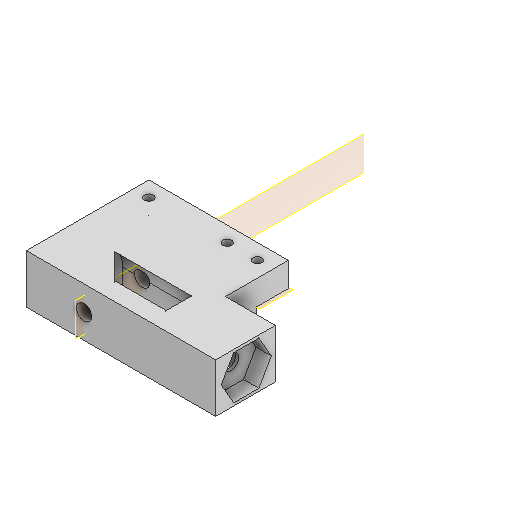
# Autodesk Inventor part: 30_Lightsheet_generator_passive_lid_v0
Saved by Autodesk Inventor 2022 (Build 260153000, 153)
## iProperties
Created: 2022-12-16
Part Number: 30_Lightsheet_generator_passive_lid_v0
Material: Generisch
Document SubType Name: Modeling
Designer: UC2
Density: 1 g/cm^3
Appearance: Vorgabe
Author: UC2
Autodesk Inventor part; units mm, degrees
ref_plane "Arbeitsebene6" through (18.9, 3.95, -31.1) normal (0, 1, 0) x (-1, 0, 0)
sketch "Skizze13" plane through (18.9, 3.95, -31.1) normal (0, 1, 0) x (-1, 0, 0)
  circle A0 centre (40.5, 5) radius 1.45 projected
  line L0 (29.1796, 0.9) -> (29.1796, 0) projected
  line L1 (45.5, 0) -> (29.1796, 0) projected
  line L2 (45.5, 0) -> (45.5, 10) projected
  line L3 (45.5, 10) -> (29.1796, 10) projected
  line L4 (29.1796, 10) -> (29.1796, 6.8717) projected
  line L5 (29.1796, 6.8717) -> (32.9296, 6.8717) projected
  line L6 (32.9296, 6.8717) -> (32.9296, 0.9) projected
  line L7 (32.9296, 0.9) -> (29.1796, 0.9) projected
  line L8 (24.1796, 0) -> (24.1796, 0.9) projected
  line L9 (24.1796, 0.9) -> (20.4296, 0.9) projected
  line L10 (20.4296, 0.9) -> (20.4296, 6.8717) projected
  line L11 (20.4296, 6.8717) -> (24.1796, 6.8717) projected
  line L12 (24.1796, 6.8717) -> (24.1796, 10) projected
  line L13 (24.1796, 10) -> (0, 10) projected
  line L14 (0, 0) -> (0, 10) projected
  line L15 (24.1796, 0) -> (0, 0) projected
  circle A1 centre (14.9199, 5) radius 1.45 projected
  circle A2 centre (5.0801, 5) radius 1.45 projected
  line L16 (29.1796, 10) -> (24.1796, 10)
  line L17 (29.1796, 0) -> (24.1796, 0)
  line L18 (55.5, 0) -> (55.5, 10) projected
  line L19 (55.5, 10) -> (55.473, 10) projected
  line L20 (55.473, 10) -> (55.473, 40) projected
  line L21 (55.473, 40) -> (45.5, 40) projected
  line L22 (45.5, 40) -> (45.5, 20) projected
  line L23 (45.5, 20) -> (35.5, 20) projected
  line L24 (35.5, 20) -> (35.5, 10.0274) projected
  arc A3 (35.5, 10.0274) -> (35.527, 10) centre (40.5, 14.9264) ccw projected
  line L25 (45.5, 10) -> (35.527, 10) projected
  line L26 (45.5, 0) -> (45.5, 10) projected
  line L27 (45.5, 0) -> (55.5, 0) projected
  line L28 (52.073, 16.5) -> (52.073, 3.5) projected
  arc A4 (48.873, 3.5) -> (52.073, 3.5) centre (50.473, 3.5) ccw projected
  line L29 (48.873, 3.5) -> (48.873, 16.5) projected
  arc A5 (52.073, 16.5) -> (48.873, 16.5) centre (50.473, 16.5) ccw projected
  line L30 (48.8865, 23.1111) -> (48.8865, 36.1111) projected
  arc A6 (52.0865, 36.1111) -> (48.8865, 36.1111) centre (50.4865, 36.1111) ccw projected
  line L31 (52.0865, 36.1111) -> (52.0865, 23.1111) projected
  arc A7 (48.8865, 23.1111) -> (52.0865, 23.1111) centre (50.4865, 23.1111) ccw projected
  line L32 (-10, 0) -> (0, 0) projected
  line L33 (0, 10) -> (0, 0) projected
  line L34 (16, 10) -> (0, 10) projected
  line L35 (16, 10) -> (16, 20) projected
  line L36 (16, 20) -> (-10, 20) projected
  line L37 (-10, 20) -> (-10, 0) projected
  line L38 (-3.4, 16.5) -> (-3.4, 3.5) projected
  arc A8 (-6.6, 3.5) -> (-3.4, 3.5) centre (-5, 3.5) ccw projected
  line L39 (-6.6, 3.5) -> (-6.6, 16.5) projected
  arc A9 (-3.4, 16.5) -> (-6.6, 16.5) centre (-5, 16.5) ccw projected
  line L40 (-16.2879, 40) -> (45.5, 40)
  line L41 (45.5, 40) -> (45.5, 20.5)
  line L42 (45.5, 20.5) -> (-16.2879, 20.5)
  line L43 (-16.2879, 20.5) -> (-16.2879, 40)
  line L44 (45.5, 20.5) -> (35.5, 20.5)
  line L45 (35.5, 20.5) -> (35.5, 20)
  line L46 (35.5, 20) -> (45.5, 20)
  line L47 (45.5, 20) -> (45.5, 20.5)
  line L48 (16, 20) -> (0, 20)
  line L49 (0, 20) -> (0, 20.5)
  line L50 (0, 20.5) -> (16, 20.5)
  line L51 (16, 20.5) -> (16, 20)
  line L52 (0, 20) -> (0, 10)
  line L53 (35.5, 10) -> (45.5, 10)
  line L54 (45.5, 10) -> (45.5, 20.5)
  line L55 (45.5, 20.5) -> (35.5, 20.5)
  line L56 (35.5, 20.5) -> (35.5, 10)
  point P0 (0, 20)
  point P1 (0.5252, 10)
  point P2 (35.527, 10)
  point P3 (0, 20)
  point P4 (35.5, 10.0274)
  dimension "d60" = 0.5
  constraints: 38 end point, 9 parallel, 5 horizontal, 5 perpendicular, 3 point on line
  measures "d60" distance between parallel lines of L23 L42
extrude "Extrusion12" add sketch "Skizze13" along normal blind 8 contours L7 L6 L5 L4 L3 L2 L1 L0 | L0 L17 L8 L9 L10 L11 L12 L16 L4 L5 L6 L7 | L15 L14 L13 L12 L11 L10 L9 L8 | L3 A3 L24 L23 L54 | L23 L45 L42 L22 | L52 L36 L35 L13 | L16 L13 L35 L51 L42 L45 L24 L56 L3 | L42 L43 L40 L22 | L49 L42 L51 L36
sketch "Skizze16" plane through (18.9, 3.95, -31.1) normal (0, -1, 0) x (1, 0, 0)
  line L0 (16.2879, 20.5) -> (0, 20.5) projected
  line L1 (-45.5, 0) -> (-45.5, 40) projected
  circle A0 centre (-5.0801, 5) radius 1.45 projected
  circle A1 centre (-14.9199, 5) radius 1.45 projected
  line L2 (-16, 20) -> (10, 20) projected
  line L3 (-66.9798, -10.3003) -> (9.2505, 65.9301)
  line L4 (16.2879, 20.5) -> (0, 20.5) projected
  line L5 (16.2879, 20.5) -> (-45.5, 20.5)
  line L6 (-45.5, 20.5) -> (-45.5, 40)
  line L7 (-45.5, 40) -> (16.2879, 40)
  line L8 (16.2879, 40) -> (16.2879, 20.5)
  line L9 (0, 20.5) -> (0, 0) projected
  line L10 (16.2879, 40) -> (16.2879, 20.5) projected
  line L11 (-45.5, 40) -> (16.2879, 40) projected
  line L12 (0, 0) -> (-45.5, 0) projected
  point P0 (-18.9, 31.1)
  constraints: 10 end point, 2 parallel, 1 horizontal, 1 perpendicular, 3 other
extrude "Extrusion13" add sketch "Skizze16" along normal blind 8 contours L0 L5 L3 L7 L8 | L5 L1 L7 L3
ref_plane "Arbeitsebene7" through (-7.7796, -1.85, -37.9251) normal (1, 0, 0) x (0, -1, 0)
sketch "Skizze18" plane through (-7.7796, -1.85, -37.9251) normal (1, 0, 0) x (0, -1, 0)
  arc A0 (-5.8, -13.6968) -> (-0.7, -9.8391) centre (-5.8, -8.3968) ccw projected
  line L0 (-0.7, -9.8391) -> (-0.7, -7.7251) projected
  arc A1 (-10.8, -9.8251) -> (-0.8, -9.8251) centre (-5.8, -8.3968) ccw projected
  line L1 (-0.8, -7.8251) -> (-0.8, -9.8251) projected
  line L2 (-10.8, -7.8251) -> (-0.8, -7.8251) projected
  line L3 (-10.8, -9.8251) -> (-10.8, -7.8251) projected
  arc A2 (-10.9, -9.8391) -> (-0.7, -9.8391) centre (-5.8, -8.3968) ccw
  line L4 (-10.9, -9.8391) -> (-10.9, -7.7251)
  line L5 (-10.9, -7.7251) -> (-0.7, -7.7251)
  line L6 (-0.7, -7.7251) -> (-0.7, -9.8391)
  point P0 (-1.85, -37.9251)
  point P1 (-5.8, -13.6968)
  constraints: 6 end point, 2 point on circle, 1 centre point, 3 other
extrude "Extrusion15" cut sketch "Skizze18" along normal mid plane 12.5 contours A2 L4 L5 L0 A0 | L3 L2 L1 A1
sketch "Skizze19" plane through (35.1879, 11.95, 8.9) normal (1, 0, 0) x (0, 0, -1)
  circle A0 centre (10, -8) radius 7 projected
  circle A1 centre (10, -8) radius 7.1
  line L0 (14.0992, -15.1) -> (5.9008, -15.1)
  line L1 (5.9008, -15.1) -> (1.8016, -8)
  line L2 (1.8016, -8) -> (5.9008, -0.9)
  line L3 (5.9008, -0.9) -> (14.0992, -0.9)
  line L4 (14.0992, -0.9) -> (18.1984, -8)
  line L5 (18.1984, -8) -> (14.0992, -15.1)
  line L6 (19.5, -16) -> (0, -16) projected
  point P0 (8.9, -11.95)
  dimension "d68" = 0.1
  constraints: 12 end point, 1 centre point, 1 coincident, 1 parallel, 1 tangent, 13 other
  measures "d68" radial gap between concentric circles of A0 A1
ref_plane "Arbeitsebene8" through (22.1204, -2.15, -7.2) normal (1, 0, 0) x (0, 1, 0)
extrude "Extrusion16" cut sketch "Skizze19" against normal blind 5 contours A0 | A1 | A1 L4 L5 | A1 L3 L4 | L5 L0 A1 | A1 L2 L3 | L0 L1 A1 | A1 L1 L2
sketch "Skizze20" plane through (30.1879, 11.05, 2.9992) normal (1, 0, 0) x (0, 0, -1)
  arc A0 (6.1223, -12.104) -> (2.4773, -12.2481) centre (4.0992, -7.1) ccw projected
  circle A1 centre (4.0992, -7.1) radius 6.15
  line L0 (10.2492, -7.1) -> (-2.0508, -7.1)
  line L1 (-2.0508, -7.1) -> (-2.0508, -16.2052)
  line L2 (-2.0508, -16.2052) -> (10.2492, -16.2052)
  line L3 (10.2492, -16.2052) -> (10.2492, -7.1)
  point P0 (2.9992, -11.05)
  point P1 (-2.0508, -7.1)
  dimension "d71" = 12.3
  constraints: 8 end point, 2 parallel, 1 coincident, 1 horizontal, 1 perpendicular, 3 other
ref_plane "Arbeitsebene9" through (-36.7921, -9.8415, -30.1125) normal (-0.7071, 0, 0.7071) x (0.7071, 0, 0.7071)
extrude "Extrusion17" cut sketch "Skizze20" against normal up to surface surface through (-36.7921, -9.8415, -30.1125) normal (-0.7071, 0, 0.7071)
ref_plane "Arbeitsebene10" through (13.1879, 11.05, 2.9992) normal (-1, 0, 0) x (0, 0, 1)
sketch "Skizze21" plane through (13.1879, 11.05, 2.9992) normal (-1, 0, 0) x (0, 0, 1)
  arc A0 (-3.1969, -9.9981) -> (-5.2274, -9.9178) centre (-4.0992, -7.1) ccw projected
  circle A1 centre (-4.0992, -7.1) radius 9
  line L0 (-13.0992, -7.1) -> (4.9008, -7.1)
  line L1 (4.9008, -7.1) -> (4.9008, -20.07)
  line L2 (4.9008, -20.07) -> (-13.0992, -20.07)
  line L3 (-13.0992, -20.07) -> (-13.0992, -7.1)
  point P0 (-2.9992, -11.05)
  dimension "d75" = 18
  constraints: 8 end point, 2 parallel, 2 point on circle, 1 centre point, 1 coincident, 1 horizontal, 1 perpendicular
  measures "d75" diameter of A1
ref_plane "Arbeitsebene11" through (-36.7921, -9.8415, -30.1125) normal (-0.7071, 0, 0.7071) x (0.7071, 0, 0.7071)
extrude "Extrusion18" cut sketch "Skizze21" along normal up to surface surface through (-36.7921, -9.8415, -30.1125) normal (-0.7071, 0, 0.7071)
sketch "Skizze22" plane through (18.9, -4.05, -31.1) normal (0, -1, 0) x (1, 0, 0)
  line L0 (-45.5, 20.5) -> (16.2879, 20.5) projected
  line L1 (-45.5, 40) -> (-45.5, 20.5) projected
  line L2 (-34.6684, 23.7083) -> (-19.8191, 38.5575)
  line L3 (-19.8191, 38.5575) -> (-18.9706, 37.709)
  line L4 (-18.9706, 37.709) -> (-33.8198, 22.8597)
  line L5 (-33.8198, 22.8597) -> (-34.6684, 23.7083)
  line L6 (-34.6684, 23.7083) -> (-18.9706, 37.709) construction
  line L7 (-19.8191, 38.5575) -> (-33.8198, 22.8597) construction
  line L8 (-34.6684, 23.7083) -> (-13.6684, 23.7083) construction
  line L9 (16.2879, 40) -> (-45.5, 40) projected
  line L10 (16.2879, 20.5) -> (16.2879, 40) projected
  point P0 (-18.9, 31.1)
  point P1 (-26.8195, 30.7086)
  dimension "d78" = 21
  dimension "d79" = 45
  dimension "d80" = 1.2
  constraints: 14 end point, 2 midpoint, 2 parallel, 1 equal length, 1 horizontal, 1 perpendicular
  measures "d78" distance of L2.start L2.end
  measures "d79" angle of L8 L2
  measures "d80" distance of L2.end L3.end
extrude "Extrusion19" cut sketch "Skizze22" against normal blind 14 contours L2 L3 L4 L5
sketch "Skizze23" plane through (18.9, -4.05, -31.1) normal (0, -1, 0) x (1, 0, 0)
  line L0 (-45.5, 20.5) -> (16.2879, 20.5) projected
  line L1 (-45.5, 40) -> (-45.5, 20.5) projected
  line L2 (-35.6796, 21) -> (-32.9713, 23.7083)
  line L3 (-33.3878, 23.2918) -> (-30.8027, 25.8769) projected
  line L4 (-5.7121, 21) -> (-35.6796, 21) projected
  line L5 (-32.9713, 21) -> (-32.9713, 23.7083)
  line L6 (-18.9706, 37.709) -> (-19.9714, 36.7082) projected
  line L7 (-19.9714, 36.7082) -> (-17.0744, 36.7082)
  line L8 (-17.0744, 36.7082) -> (-17.0744, 39)
  line L9 (-18.9706, 37.709) -> (-19.9714, 36.7082) projected
  line L10 (-19.9714, 36.7082) -> (-17.6796, 39)
  line L11 (-17.6796, 39) -> (-17.0744, 39)
  line L12 (16.2879, 40) -> (-45.5, 40) projected
  line L13 (16.2879, 20.5) -> (16.2879, 40) projected
  point P0 (-18.9, 31.1)
  point P1 (-29.1796, 21)
  constraints: 12 end point, 2 horizontal, 2 perpendicular, 2 point on line, 1 collinear
extrude "Extrusion20" add sketch "Skizze23" against normal up to surface (16 mm away) contours L2 L5 L4 | L10 L11 L8 L7 L6
sketch "Skizze24" plane through (30.1879, 11.95, 8.9) normal (1, 0, 0) x (0, 0, -1)
  arc A0 (16.15, -8) -> (3.85, -8) centre (10, -8) ccw projected
  circle A1 centre (10, -8) radius 2.5 projected
  circle A2 centre (10, -8) radius 6.15
  line L0 (14.0992, -0.9) -> (18.1984, -8) projected
  line L1 (18.1984, -8) -> (14.0992, -15.1) projected
  line L2 (14.0992, -15.1) -> (5.9008, -15.1) projected
  line L3 (5.9008, -15.1) -> (1.8016, -8) projected
  line L4 (1.8016, -8) -> (5.9008, -0.9) projected
  line L5 (5.9008, -0.9) -> (14.0992, -0.9) projected
  line L6 (19.5, -16) -> (19.5, 0) projected
  line L7 (0, 0) -> (19.5, 0) projected
  line L8 (0, -16) -> (0, 0) projected
  line L9 (19.5, -16) -> (0, -16) projected
  point P0 (8.9, -11.95)
  constraints: 1 centre point, 1 coincident, 1 concentric
extrude "Extrusion21" add sketch "Skizze24" against normal blind 1 contours A2 A0 | L0 L1 L2 L3 L4 L5 | L9 L8 L7 L6
ref_plane "Arbeitsebene12" through (-26.6, -8.85, -11.1) normal (1, 0, 0) x (0, 1, 0)
sketch "Skizze25" plane through (18.9, 3.95, -10.6) normal (1, 0, 0) x (0, 0, -1)
  line L0 (0.5, -6.8) -> (20.5, -6.8) projected
  line L1 (0, -8) -> (0, 8) projected
  line L2 (0, 0) -> (10.5, 0) projected
  line L3 (0, 0) -> (10, 0)
  line L4 (10, 0) -> (10, -6.8)
  line L5 (10, -6.8) -> (0, -6.8)
  line L6 (0, -6.8) -> (0, 0)
  line L7 (10.5, 0) -> (10.5, -6.8) projected
  point P0 (-10.6, -3.95)
  point P1 (0, -6.8)
  dimension "d87" = 0.5
  constraints: 8 end point, 2 parallel, 1 horizontal, 1 perpendicular, 1 point on line
  measures "d87" distance between parallel lines of L7 L4
extrude "Extrusion22" add sketch "Skizze25" against normal up to surface (45.5 mm away) contours L5 L1 L2 L4 L0
sketch "Skizze26" plane through (18.9, 11.95, -31.1) normal (0, 0, -1) x (-1, 0, 0)
  line L0 (0, -8) -> (24.1796, -8) projected
  line L1 (0, 0) -> (24.1796, 0) projected
  line L2 (0, -8) -> (0, 0) projected
  line L3 (24.1796, -8) -> (29.1796, -8) projected
  circle A0 centre (26.6796, -8) radius 2.5
  line L4 (24.1796, -8) -> (24.1796, 0) projected
  point P0 (18.9, -11.95)
  constraints: 1 horizontal alignment, 2 other
extrude "Extrusion23" cut sketch "Skizze26" against normal through all contours A0 L3 | L3 A0
